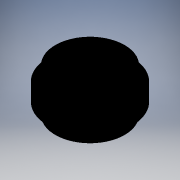
# Autodesk Inventor part: HFROLL5_b
Saved by Autodesk Inventor 2017.3 (Build 213256000, 256)
## iProperties
Part Number: HFROLL5_b
Material: Generic
Catalog Web Link: www.cadenas.de
Description: HFROLL, HFROLLM_body-Rollers for Aluminum Frames
Vendor: MISUMI
Document SubType Name: Modeling
Designer: partserver
Manufacturer: MISUMI
Mass: 7.03748 g
Surface Area: 28.4685 cm^2
Volume: 7.03748 cm^3
Density: 1 g/cm^3
Appearance: PSOLRGB-192-192-192
Category: PARTsolutions
Company: MISUMI
Title: HFROLL5
Author: Cadenas PARTsolutions
Comments: Rollers for Aluminum Frames
PSOL_IDENT_0: {$CADENAS_DATA\23d-libs\misumi\metric\39_accessories_for_al_extrusions\hfroll\hfroll_body.prj},175 {
PSOL_IDENT_1: VTYP=3D},{NB=HFROLL5_b},{LINA=HFROLL5},{NN=HFROLL, HFROLLM_body},{DATE=30.03.2018 07:06:35},{GEOMDAT
PSOL_IDENT_2: E=10.06.2016 08:25:00},{VERSION=},{LINEID=10},{WBVAR=MATAC},{WBNUMERIC=}  {NB=HFROLL5_b},{LINA=HFROL
PSOL_IDENT_3: L5},{KT=DUMMY},{PN=HFROLL5},{MATAC=HFROLL},{MATR=Nylon 6},{TYPE=HFROLL},{NO=5},{CFSW=6},{CFT=20-40 S
PSOL_IDENT_4: q.},{H=6.0},{D=24},{T=15.0},{TT1=4},{TT2=5},{DD1=29.0},{DD2=9.2},{COLOR=Black},{BEARING=None},{ACL=1
PSOL_IDENT_5: 6.5},{ACTT3=1.5},{ACD2=9},{ACDD4=6.2},{ACDD5=13},{QAC=1}
NB: HFROLL5_b
NN: HFROLL, HFROLLM_body
NT: Rollers for Aluminum Frames
NBSYN: $PN._b
LINA: HFROLL5
CATALOG: Misumi
MATAC: Nylon 6
MATR: Nylon 6
NO: 5
CFSW: 6
CFT: 20-40 Sq.
H: 6
D: 24
T: 15
TT1: 4
TT2: 5
DD1: 29
DD2: 9.2
COLOR: Black
ACL: 16.5
ACTT3: 1.5
ACD2: 9
ACDD4: 6.2
ACDD5: 13
QAC: 1
SUPPLIER: MISUMI
ARTICLENO: HFROLL5_b
BOMINFO: HFROLL5
CREATOR: CADENAS GmbH
Autodesk Inventor part; units mm, degrees
sketch "Sketch_1" plane through (0, 0, 0) normal (1, 0, 0) x (0, 1, 0)
  line L0 (0, -7.5) -> (0, 7.5)
  line L1 (4.6, 7.5) -> (4.6, -7.5)
  line L2 (4.6, -7.5) -> (12, -7.5)
  line L3 (12, -7.5) -> (12, -2.5)
  line L4 (12, -2.5) -> (14.5, -2.5)
  line L5 (14.5, -2.5) -> (14.5, 3.5)
  line L6 (14.5, 3.5) -> (12, 3.5)
  line L7 (12, 3.5) -> (12, 7.5)
  line L8 (12, 7.5) -> (4.6, 7.5)
  constraints: 18 end point
revolve "Revolution1" add sketch "Sketch_1" angle 360 about axis through (0, 0, -7.5) along (0, 0, -1)
ref_plane "1_XY" through (0, 0, -7.5) normal (0, 0, 1) x (1, 0, 0)
ref_plane "1_YZ" through (0, 0, -7.5) normal (1, 0, 0) x (0, 1, 0)
ref_plane "1_ZX" through (0, 0, -7.5) normal (0, 1, 0) x (0, 0, 1)
ref_plane "2_XY" through (0, 0, 7.5) normal (0, 0, 1) x (1, 0, 0)
ref_plane "2_YZ" through (0, 0, 7.5) normal (1, 0, 0) x (0, 1, 0)
ref_plane "2_ZX" through (0, 0, 7.5) normal (0, 1, 0) x (0, 0, 1)
body "Solid1"
